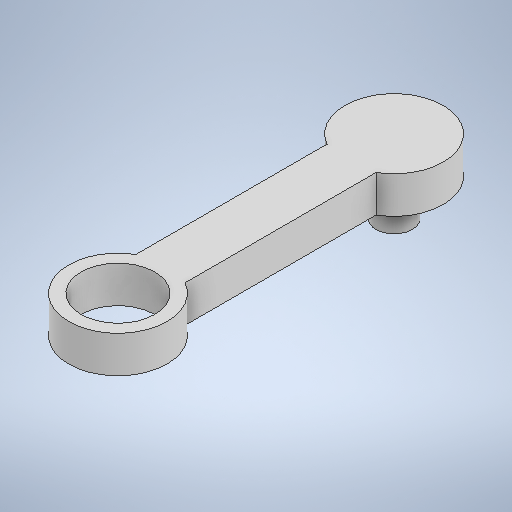
# Autodesk Inventor part: 204
Saved by Autodesk Inventor 2025.1 (Build 291241000, 241)
## iProperties
Created: 2024-09-02
Part Number: 204
Material: Generisch
Document SubType Name: Modeling
Designer: ffogue
Density: 1 g/cm^3
Appearance: Vorgabe
Author: ffogue
Autodesk Inventor part; units mm, degrees
ref_plane "YZ Plane" through (0, 0, 0) normal (1, 0, 0) x (0, 1, 0)
ref_plane "XZ Plane" through (0, 0, 0) normal (0, 1, 0) x (-1, 0, 0)
ref_plane "XY Plane" through (0, 0, 0) normal (0, 0, 1) x (1, 0, 0)
sketch "Sketch1" plane through (0, 0, 0) normal (0, 0, 1) x (1, 0, 0)
  arc A0 (-4, -15.5718) -> (4, -15.5718) centre (0, -22.5) ccw
  arc A1 (4, 15.5718) -> (-4, 15.5718) centre (0, 22.5) ccw
  line L0 (-4, 15.5718) -> (-4, -15.5718)
  line L1 (4, 15.5718) -> (4, -15.5718)
  circle A2 centre (0, 22.5) radius 3
  circle A3 centre (0, -22.5) radius 6
  point P0 (0, 0)
  dimension "d0" = 45
  dimension "d1" = 22.5
  dimension "d2" = 8
  dimension "d3" = 4
  dimension "d6" = 8
  dimension "d7" = 8
  dimension "d8" = 12
  dimension "d9" = 6
  constraints: 4 centre point, 4 end point, 4 point on circle, 2 coincident, 2 horizontal alignment, 2 vertical, 2 vertical alignment
  measures "d0" distance of A0.centre A1.centre
  measures "d1" distance of A0.centre point (0, 0)
  measures "d2" distance between parallel lines of L1 L0
  measures "d3" distance from line of L0 point (0, 0)
  measures "d6" radius of A1
  measures "d7" radius of A0
  measures "d8" diameter of A3
  measures "d9" diameter of A2
extrude "Extrusion1" add sketch "Sketch1" against normal blind 6
extrude "Extrusion2" add sketch "Sketch1" against normal blind 12 contours A2
equation "\"d1\" = 0.5 * d0"
body "Solid1"
